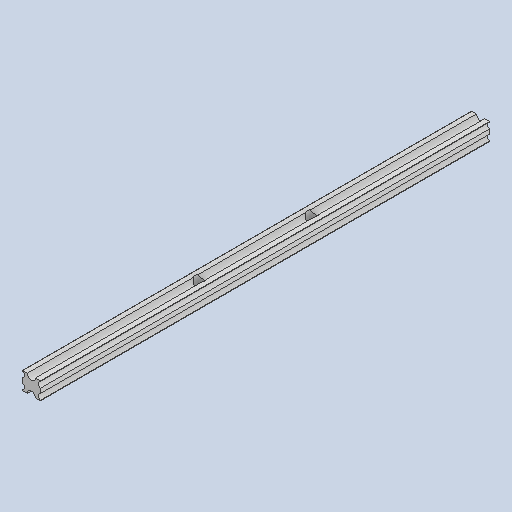
# Autodesk Inventor part: KC-362-30 Middle
Saved by Autodesk Inventor 2022 (Build 260153000, 153)
## iProperties
Created: 2021-09-24
Part Number: KC-362-30 Middle
Material: Generic
Document SubType Name: Modeling
Designer: deli
Density: 1 g/cm^3
Appearance: Default
Author: deli
Autodesk Inventor part; units mm, degrees
ref_plane "YZ Plane" through (0, 0, 0) normal (1, 0, 0) x (0, 1, 0)
ref_plane "XZ Plane" through (0, 0, 0) normal (0, 1, 0) x (-1, 0, 0)
ref_plane "XY Plane" through (0, 0, 0) normal (0, 0, 1) x (1, 0, 0)
sketch "Sketch1" plane through (0, 0, 0) normal (0, 0, 1) x (1, 0, 0)
  line L0 (12, 5.8) -> (8.75, 5.8) projected
  arc A0 (3.25, 5.8) -> (8.75, 5.8) centre (6, 5.8) ccw projected
  line L1 (3.25, 5.8) -> (0, 5.8) projected
  arc A1 (0, 1.5201) -> (0, 5.4799) centre (-0.7, 3.5) ccw projected
  line L2 (0, 1.5201) -> (0, -1.5201) projected
  arc A2 (0, -5.4799) -> (0, -1.5201) centre (-0.7, -3.5) ccw projected
  line L3 (0, -5.8) -> (3.25, -5.8) projected
  arc A3 (8.75, -5.8) -> (3.25, -5.8) centre (6, -5.8) ccw projected
  line L4 (8.75, -5.8) -> (12, -5.8) projected
  arc A4 (12, -1.5201) -> (12, -5.4799) centre (12.7, -3.5) ccw projected
  line L5 (12, -5.8) -> (12, -5.4799) projected
  line L6 (12, -1.5201) -> (12, 1.5201) projected
  arc A5 (12, 5.4799) -> (12, 1.5201) centre (12.7, 3.5) ccw projected
  line L7 (12, 5.4799) -> (12, 5.8) projected
  line L8 (0, 5.8) -> (0, 5.4799) projected
  line L9 (0, -5.4799) -> (0, -5.8) projected
  point P0 (0, 0)
extrude "Extrusion1" add sketch "Sketch1" against normal blind 300
sketch "Sketch2" plane through (12, 5.8, 0) normal (0, 1, 0) x (1, 0, 0)
  arc A0 (-8.75, 189.2321) -> (-8.75, 185.7679) centre (-6, 187.5) ccw projected
  arc A1 (-8.75, 114.2321) -> (-8.75, 110.7679) centre (-6, 112.5) ccw projected
  circle A2 centre (-6, 187.5) radius 3.25
  circle A3 centre (-6, 112.5) radius 3.25
  point P0 (-12, 0)
  point P1 (-8.75, 110.7679)
  point P2 (-8.75, 114.2321)
  point P3 (-8.75, 185.7679)
  constraints: 2 centre point, 2 coincident, 2 concentric
extrude "Extrusion2" cut sketch "Sketch2" against normal blind 300
body "Solid1"
